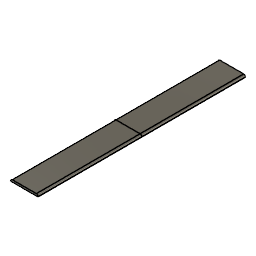
casomira-semafor-suplik-dlouhý (Autodesk Fusion 360 design; units mm, degrees)
Autodesk Fusion 360 part; units mm, degrees
sketch "Sketch1" plane through (0, 0, 0) normal (0, 0, 1) x (1, 0, 0)
  line L0 (0, 0) -> (39.9, 0)
  line L1 (39.9, 0) -> (39.9, 150)
  line L2 (39.9, 150) -> (0, 150)
  line L3 (0, 150) -> (0, 0)
  dimension "d1" = 39.9
  dimension "d2" = 150
  constraint horizontal L0
  constraint vertical L1
  constraint horizontal L2
  constraint vertical L3
  constraint coincident L0.start L3.end
  measures "d1" distance of L0.start L0.end
  measures "d2" distance of L0.start L2.end
extrude "Extrude1" add sketch "Sketch1" along normal blind 2.98 makes body 1
fillet "Fillet1" radius 2.5 2 edges at (39.9, 75, 2.98) (0, 75, 2.98) on bodies 1
mirror "Mirror1" about plane through (39.9, 150, 0) normal (0, 1, 0) of bodies 1 makes body 2
